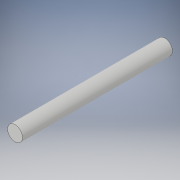
# Autodesk Inventor part: motoradaptor
Saved by Autodesk Inventor 2018 (Build 220112000, 112)
## iProperties
Created: 2019-05-01
Part Number: motoradaptor
Material: Generic
Document SubType Name: Modeling
Designer: F8PLTW
Density: 1 g/cm^3
Appearance: Default
Author: F8PLTW
Autodesk Inventor part; units mm, degrees
ref_plane "YZ Plane" through (0, 0, 0) normal (1, 0, 0) x (0, 1, 0)
ref_plane "XZ Plane" through (0, 0, 0) normal (0, 1, 0) x (-1, 0, 0)
ref_plane "XY Plane" through (0, 0, 0) normal (0, 0, 1) x (1, 0, 0)
sketch "Sketch1" plane through (0, 0, 0) normal (0, 0, 1) x (1, 0, 0)
  circle A0 centre (-0.9126, 2.0208) radius 3.175
  circle A1 centre (-0.9126, 2.0208) radius 6.35
  point P0 (0, 0)
  dimension "d0" = 6.35
  dimension "d1" = 12.7
  constraints: 2 centre point, 1 coincident
  measures "d0" diameter of A0
  measures "d1" diameter of A1
extrude "Extrusion1" add sketch "Sketch1" along normal blind 25.4
sketch "Sketch2" plane through (-0.9126, 2.0208, 25.4) normal (0, 0, 1) x (1, 0, 0)
  line L0 (-3.2261, 4.7402) -> (3.0392, 4.7402)
  line L1 (3.0392, 4.7402) -> (3.0392, 2.5812)
  line L2 (3.0392, 2.5812) -> (-3.2261, 2.5812)
  line L3 (-3.2261, 2.5812) -> (-3.2261, 4.7402)
  point P0 (0.9126, -2.0208)
  dimension "d6" = 2.159
  constraints: 8 end point, 2 parallel, 1 horizontal, 1 perpendicular
  measures "d6" distance of L0.end L1.end
extrude "Extrusion2" add sketch "Sketch2" against normal blind 25.4
sketch "Sketch3" plane through (-0.9126, 2.0208, 25.4) normal (0, 0, 1) x (1, 0, 0)
  circle A0 centre (0, 0) radius 6.35
  point P0 (0.9126, -2.0208)
  constraints: 1 centre point
extrude "Extrusion3" add sketch "Sketch3" along normal blind 101.6
body "Solid1"
